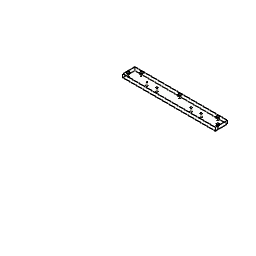
CAD_File 14 (Autodesk Fusion 360 design; units mm, degrees)
Autodesk Fusion 360 part; units mm, degrees
sketch "Sketch1" plane through (0, 0, 192) normal (0, 0, 1) x (-1, 0, 0)
  line L0 (115, 107) -> (107, 107)
  line L1 (107, -107) -> (115, -107)
  line L2 (115, -107) -> (115, 107)
  line L3 (115, -115) -> (-115, -115)
  line L4 (-115, -115) -> (-115, -85)
  line L5 (115, -85) -> (-115, -85)
  line L6 (115, -85) -> (115, -115)
  dimension "d774" = 115
  dimension "d775" = 30
  constraint horizontal L3
  constraint vertical L4
  constraint coincident L2 L5.start
  constraint perpendicular L4 L5
  measures "d774" distance of origin L3
  measures "d775" distance of L3 L5
extrude "Extrude1" add sketch "Sketch1" along normal blind 8
sketch "Sketch3" plane through (0, 0, 200) normal (0, 0, 1) x (-1, 0, 0)
  line L0 (115, -85) -> (-115, -85)
  line L1 (-115, -85) -> (-115, -115)
  line L2 (-115, -115) -> (115, -115)
  line L3 (115, -115) -> (115, -85)
  circle A0 centre (67.507, -27.4968) radius 2.75
  circle A1 centre (42.5642, -27.4968) radius 2.75
  circle A2 centre (-42.5642, -27.4968) radius 2.75
  circle A3 centre (-67.507, -27.4968) radius 2.75
  circle A4 centre (-42.5642, -27.4968) radius 2.5
  circle A5 centre (-67.507, -27.4968) radius 2.5
  circle A6 centre (42.5642, -27.4968) radius 2.5
  circle A7 centre (67.507, -27.4968) radius 2.5
  dimension "d800" = 5
  dimension "d801" = 5
  dimension "d802" = 5
  dimension "d803" = 5
  constraint concentric A2 A4
  constraint concentric A3 A5
  constraint concentric A1 A6
  constraint concentric A0 A7
  measures "d800" diameter of A4
  measures "d801" diameter of A5
  measures "d802" diameter of A6
  measures "d803" diameter of A7
extrude "Extrude6" cut sketch "Sketch3" against normal up to surface (8 mm away) contours A4 | A5 | A6 | A7
sketch "Sketch4" plane through (0, 0, 200) normal (0, 0, 1) x (-1, 0, 0)
  line L0 (115, -85) -> (-115, -85)
  line L1 (-115, -85) -> (-115, -115)
  line L2 (-115, -115) -> (115, -115)
  line L3 (115, -115) -> (115, -85)
  circle A0 centre (-67.507, -97.4968) radius 2.75
  circle A1 centre (-42.5642, -97.4968) radius 2.75
  circle A2 centre (42.5642, -97.4968) radius 2.75
  circle A3 centre (67.507, -97.4968) radius 2.75
  circle A4 centre (67.507, -97.4968) radius 2.5
  circle A5 centre (42.5642, -97.4968) radius 2.5
  circle A6 centre (-42.5642, -97.4968) radius 2.5
  circle A7 centre (-67.507, -97.4968) radius 2.5
  dimension "d846" = 5
  dimension "d847" = 5
  dimension "d848" = 5
  dimension "d849" = 5
  constraint concentric A3 A4
  constraint concentric A2 A5
  constraint concentric A1 A6
  constraint concentric A0 A7
  measures "d846" diameter of A4
  measures "d847" diameter of A5
  measures "d848" diameter of A6
  measures "d849" diameter of A7
extrude "Extrude7" cut sketch "Sketch4" against normal blind 8 contours A4 | A5 | A6 | A7
thread "Thread2" "ISO Metric profile 5.0 M5x0.8 6H" major diameter 5.12 minor diameter 4.234 pitch 0.8 angle 60 resizes the face on face at (-69.8107, 96.5257, 194.6667) on face at (45.0518, 97.7457, 194.6667) on face at (-45.0518, 97.7457, 197.3333) on face at (69.8107, 98.4679, 194.6667)
sketch "Sketch5" plane through (0, 0, 200) normal (0, 0, 1) x (-1, 0, 0)
  circle A0 centre (-42.5642, -97.4968) radius 2.117
  circle A1 centre (67.507, -97.4968) radius 2.117
  circle A2 centre (-67.507, -97.4968) radius 2.117
  circle A3 centre (42.5642, -97.4968) radius 2.117
  line L0 (115, -85) -> (-115, -85)
  line L1 (-115, -85) -> (-115, -115)
  line L2 (-115, -115) -> (115, -115)
  line L3 (115, -115) -> (115, -85)
  line L4 (0, -125) -> (0, -80.7797) construction
  circle A4 centre (95, -111) radius 1.5
  circle A5 centre (111, -95) radius 1.5
  circle A6 centre (0, -111) radius 1.5
  circle A7 centre (0, -111) radius 3
  circle A8 centre (95, -111) radius 3
  circle A9 centre (111, -95) radius 3
  circle A10 centre (-111, -95) radius 1.5
  circle A11 centre (-111, -95) radius 3
  circle A12 centre (-95, -111) radius 1.5
  circle A13 centre (-95, -111) radius 3
  dimension "d866" = 3
  dimension "d867" = 4
  dimension "d868" = 20
  dimension "d869" = 3
  dimension "d870" = 4
  dimension "d871" = 20
  dimension "d872" = 3
  dimension "d873" = 4
  dimension "d874" = 6
  dimension "d875" = 6
  dimension "d876" = 6
  constraint perpendicular L0 L4
  constraint coincident L4 A6.centre
  constraint concentric A6 A7
  constraint concentric A4 A8
  constraint concentric A5 A9
  constraint symmetric L4 A4 A12
  constraint symmetric L4 A5 A10
  constraint symmetric L4 A8 A13
  constraint symmetric L4 A9 A11
  measures "d866" diameter of A4
  measures "d867" distance of L2 A4.centre
  measures "d868" distance of L3 A4.centre
  measures "d869" diameter of A5
  measures "d870" distance of L3 A5.centre
  measures "d871" distance of L2 A5.centre
  measures "d872" diameter of A6
  measures "d873" distance of L2 A6.centre
  measures "d874" diameter of A7
  measures "d875" diameter of A8
  measures "d876" diameter of A9
extrude "Extrude8" cut sketch "Sketch5" against normal blind 18 contours A4 | A5 | A6 | A10 | A12
extrude "Extrude9" cut sketch "Sketch5" against normal blind 3 contours A7 | A8 | A9 | A11 | A13
